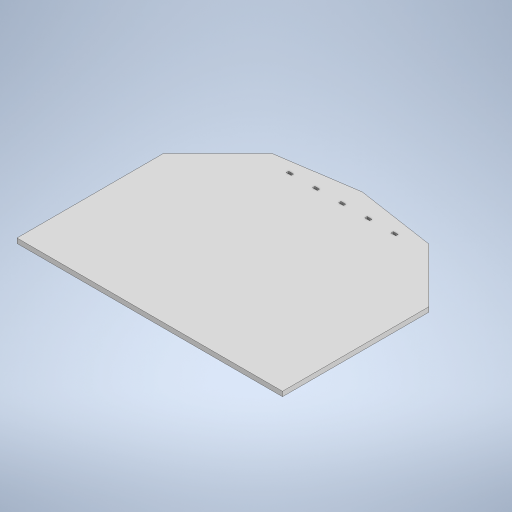
# Autodesk Inventor part: ChannelInsert
Saved by Autodesk Inventor 2023 (Build 270158000, 158)
## iProperties
Created: 2023-05-02
Part Number: ChannelInsert
Material: Generic
Document SubType Name: Modeling
Designer: 1roweste
Density: 1 g/cm^3
Appearance: Default
Author: 1roweste
Autodesk Inventor part; units mm, degrees
ref_plane "YZ Plane" through (0, 0, 0) normal (1, 0, 0) x (0, 1, 0)
ref_plane "XZ Plane" through (0, 0, 0) normal (0, 1, 0) x (-1, 0, 0)
ref_plane "XY Plane" through (0, 0, 0) normal (0, 0, 1) x (1, 0, 0)
sketch "Sketch1" plane through (0, 0, 0) normal (0, 1, 0) x (-1, 0, 0)
  line L0 (0, 2) -> (-5.5, 2)
  line L1 (-5.5, -125.4) -> (-5.5, 2)
  line L2 (0, -125.4) -> (-5.5, -125.4)
  line L3 (0, -125.4) -> (0, -123.4)
  line L4 (0, -123.4) -> (65.1, -123.4)
  line L5 (65.1, -122.5716) -> (65.1, -123.4)
  line L6 (65.1, -122.5716) -> (88.8588, -98.8128)
  line L7 (88.8588, -98.8128) -> (84.9697, -94.9237)
  line L8 (84.9697, -94.9237) -> (61.9934, -117.9)
  line L9 (0, -117.9) -> (61.9934, -117.9)
  line L10 (0, -117.9) -> (0, -5.5)
  line L11 (0, -5.5) -> (61.9934, -5.5)
  line L12 (84.9697, -28.4763) -> (61.9934, -5.5)
  line L13 (88.8588, -24.5872) -> (84.9697, -28.4763)
  line L14 (65.1, -0.8284) -> (88.8588, -24.5872)
  line L15 (65.1, 0) -> (65.1, -0.8284)
  line L16 (0, 0) -> (65.1, 0)
  line L17 (0, 0) -> (0, 2)
  line L18 (84.9697, -28.4763) -> (84.9697, -94.9237)
  line L19 (84.6161, -94.5701) -> (61.7863, -117.4)
  line L20 (61.7863, -117.4) -> (0.5, -117.4)
  line L21 (0.5, -117.4) -> (0.5, -6)
  line L22 (0.5, -6) -> (61.7863, -6)
  line L23 (61.7863, -6) -> (84.6161, -28.8299)
  point P0 (94.5, -125.4)
  dimension "d0" = 0.5
  constraints: 48 end point, 1 vertical, 4 other
  measures "d0" distance between parallel lines of L9 L20
extrude "Extrusion1" add sketch "Sketch1" along normal blind 2 contours L18 L8 L9 L10 L11 L12
sketch "Sketch2" plane through (0, 2, 0) normal (0, 1, 0) x (1, 0, 0)
  line L0 (-61.9934, 117.9) -> (-84.9697, 94.9237) projected
  line L1 (-84.9697, 94.9237) -> (-84.9697, 28.4763) projected
  line L2 (-84.9697, 28.4763) -> (-61.9934, 5.5) projected
  line L3 (-61.9934, 5.5) -> (0, 5.5) projected
  line L4 (0, 5.5) -> (0, 117.9) projected
  line L5 (0, 117.9) -> (-61.9934, 117.9) projected
  line L6 (-84.9697, 61.7) -> (-89.9697, 61.7)
  line L7 (-89.9697, 61.7) -> (-84.9697, 28.4763)
  line L8 (-89.9697, 61.7) -> (-84.9697, 94.9237)
  point P0 (0, 0)
  dimension "d3" = 5
  constraints: 6 end point, 1 horizontal, 1 midpoint
  measures "d3" distance of L6.start L6.end
extrude "Extrusion2" add sketch "Sketch2" against normal blind 1 contours L1 L6 L8 | L1 L7 L6
sketch "Sketch3" plane through (0, 2, 0) normal (0, 1, 0) x (1, 0, 0)
  line L0 (-84.9697, 94.9237) -> (-84.9697, 28.4763)
  line L1 (-81.9697, 94.9237) -> (-81.9697, 28.4763)
  line L2 (-80.9697, 62.7) -> (-81.9697, 62.7)
  line L3 (-81.9697, 62.7) -> (-81.9697, 60.7)
  line L4 (-81.9697, 60.7) -> (-80.9697, 60.7)
  line L5 (-80.9697, 60.7) -> (-80.9697, 62.7)
  line L6 (-80.9697, 51.6253) -> (-81.9697, 51.6253)
  line L7 (-81.9697, 51.6253) -> (-81.9697, 49.6253)
  line L8 (-81.9697, 49.6253) -> (-80.9697, 49.6253)
  line L9 (-80.9697, 49.6253) -> (-80.9697, 51.6253)
  line L10 (-80.9697, 40.5507) -> (-81.9697, 40.5507)
  line L11 (-81.9697, 40.5507) -> (-81.9697, 38.5507)
  line L12 (-81.9697, 38.5507) -> (-80.9697, 38.5507)
  line L13 (-80.9697, 38.5507) -> (-80.9697, 40.5507)
  line L14 (-80.9697, 73.7747) -> (-81.9697, 73.7747)
  line L15 (-81.9697, 73.7747) -> (-81.9697, 71.7747)
  line L16 (-81.9697, 71.7747) -> (-80.9697, 71.7747)
  line L17 (-80.9697, 71.7747) -> (-80.9697, 73.7747)
  line L18 (-80.9697, 62.7) -> (-81.9697, 62.7)
  line L19 (-81.9697, 62.7) -> (-81.9697, 60.7)
  line L20 (-81.9697, 60.7) -> (-80.9697, 60.7)
  line L21 (-80.9697, 60.7) -> (-80.9697, 62.7)
  line L22 (-80.9697, 51.6253) -> (-81.9697, 51.6253)
  line L23 (-81.9697, 51.6253) -> (-81.9697, 49.6253)
  line L24 (-81.9697, 49.6253) -> (-80.9697, 49.6253)
  line L25 (-80.9697, 49.6253) -> (-80.9697, 51.6253)
  line L26 (-80.9697, 84.8493) -> (-81.9697, 84.8493)
  line L27 (-81.9697, 84.8493) -> (-81.9697, 82.8493)
  line L28 (-81.9697, 82.8493) -> (-80.9697, 82.8493)
  line L29 (-80.9697, 82.8493) -> (-80.9697, 84.8493)
  line L30 (-80.9697, 73.7747) -> (-81.9697, 73.7747)
  line L31 (-81.9697, 73.7747) -> (-81.9697, 71.7747)
  line L32 (-81.9697, 71.7747) -> (-80.9697, 71.7747)
  line L33 (-80.9697, 71.7747) -> (-80.9697, 73.7747)
  line L34 (-80.9697, 62.7) -> (-81.9697, 62.7)
  line L35 (-81.9697, 62.7) -> (-81.9697, 60.7)
  line L36 (-81.9697, 60.7) -> (-80.9697, 60.7)
  line L37 (-80.9697, 60.7) -> (-80.9697, 62.7)
  point P0 (0, 0)
  point P1 (-81.9697, 61.7)
  point P2 (-81.9697, 61.7)
  point P3 (-80.9697, 61.7)
  point P4 (-81.9697, 50.6253)
  point P5 (-80.9697, 50.6253)
  point P6 (-81.9697, 50.6253)
  point P7 (-81.9697, 39.5507)
  point P8 (-80.9697, 39.5507)
  point P9 (-81.9697, 39.5507)
  point P10 (-81.9697, 72.7747)
  point P11 (-80.9697, 72.7747)
  point P12 (-81.9697, 72.7747)
  point P13 (-81.9697, 61.7)
  point P14 (-80.9697, 61.7)
  point P15 (-81.9697, 61.7)
  point P16 (-81.9697, 50.6253)
  point P17 (-80.9697, 50.6253)
  point P18 (-81.9697, 50.6253)
  point P19 (-81.9697, 83.8493)
  point P20 (-80.9697, 83.8493)
  point P21 (-81.9697, 83.8493)
  point P22 (-81.9697, 72.7747)
  point P23 (-80.9697, 72.7747)
  point P24 (-81.9697, 72.7747)
  point P25 (-81.9697, 61.7)
  point P26 (-80.9697, 61.7)
  point P27 (-81.9697, 61.7)
  dimension "d6" = 3
  dimension "d7" = 1
  dimension "d8" = 2
  dimension "d9" = 0
  dimension "d10" = 0
  dimension "d13" = 11.0747
  dimension "d16" = 11.0747
  constraints: 76 end point, 3 midpoint, 3 parallel, 2 vertical, 1 horizontal, 1 perpendicular, 88 other
  measures "d6" distance between parallel lines of L0 L1
  measures "d7" distance of L4.end L3.end
  measures "d8" distance of L3.end L2.end
  measures "d9" distance from line of L1 point (-81.97, 61.7)
  measures "d10" vertical distance of point (-81.97, 61.7) point (-80.97, 61.7)
  measures "d13" distance of L2.start L6.start
  measures "d16" distance of L2.start L14.start
extrude "Extrusion3" cut sketch "Sketch3" against normal blind 2
body "Solid1"
